Autodesk Fusion 360 part; units mm, degrees
note: some values were not read from the file. Set by a fixed rule: which sketch regions a step uses.
(part 2 of 2)
sketch "Sketch19" plane through (0, 0, 50.8) normal (0, 0, 1) x (-1, 0, 0)
  line L0 (-511.175, 2670.175) -> (-609.6, 2670.175)
  arc A0 (-609.6, 2670.175) -> (-1344.8064, 2362.3425) centre (-609.6, 1638.3) ccw
  arc A1 (-2923.5196, 2352.9776) -> (-1344.8064, 2362.3425) centre (-2138.8294, 3144.3083) ccw
  arc A2 (-2923.5196, 2352.9776) -> (-2963.6689, 2390.6683) centre (-3632.2, 1638.3) ccw
  arc A3 (-2963.6689, 2390.6683) -> (-3715.5992, 2670.175) centre (-3671.2525, 1638.3) ccw
  line L1 (-3715.5992, 2670.175) -> (-3730.6249, 2670.175)
  line L2 (-3730.6249, 2670.175) -> (-3730.6249, 2438.5075)
  line L3 (-3730.6249, 2438.5075) -> (-3759.1999, 2438.5075)
  line L4 (-3759.1999, 2438.5075) -> (-3759.1999, 3251.2)
  line L5 (-3759.1999, 3251.2) -> (-3730.6249, 3251.2)
  line L6 (-3730.6249, 3251.2) -> (-3730.6249, 3019.425)
  line L7 (-3730.6249, 3019.425) -> (-3632.2, 3019.425)
  arc A4 (-2659.7206, 2619.009) -> (-3632.2, 3019.425) centre (-3632.2, 1638.3) ccw
  arc A5 (-2659.7206, 2619.009) -> (-1611.7429, 2625.2256) centre (-2138.8294, 3144.3083) ccw
  arc A6 (-609.6, 3044.825) -> (-1611.7429, 2625.2256) centre (-609.6, 1638.3) ccw
  line L8 (-609.6, 3044.825) -> (-511.175, 3044.825)
  line L9 (-511.175, 3044.825) -> (-511.175, 3276.173)
  line L10 (-511.175, 3276.173) -> (-482.6, 3276.173)
  line L11 (-482.6, 3276.173) -> (-482.6, 3044.825)
  line L12 (-482.6, 3044.825) -> (0, 3044.825)
  line L13 (0, 3044.825) -> (0, 3276.6)
  line L14 (0, 3276.6) -> (-609.6, 3276.6)
  arc A7 (-609.6, 3276.6) -> (-1776.8816, 2787.8567) centre (-609.6, 1638.3) ccw
  arc A8 (-2496.523, 2783.5878) -> (-1776.8816, 2787.8567) centre (-2138.8294, 3144.3083) ccw
  arc A9 (-2496.523, 2783.5878) -> (-3632.2, 3251.2) centre (-3632.2, 1638.3) ccw
  line L15 (-3632.2, 3251.2) -> (-4241.8, 3251.2)
  line L16 (-4241.8, 3251.2) -> (-4241.8, 2438.4)
  line L17 (-4241.8, 2438.4) -> (-3710.305, 2438.4)
  arc A10 (-3710.305, 838.2) -> (-3710.305, 2438.4) centre (-3671.2525, 1638.3) ccw
  line L18 (-3710.305, 838.2) -> (-3730.625, 838.2)
  line L19 (-3730.625, 838.2) -> (-3730.625, 276.225)
  line L20 (-511.175, 250.825) -> (-511.175, 838.2)
  line L21 (-511.175, 838.2) -> (-482.6, 838.2)
  line L22 (-482.6, 838.2) -> (-482.6, 606.425)
  line L23 (-482.6, 606.425) -> (0, 606.425)
  line L24 (0, 606.425) -> (0, 838.2)
  line L25 (0, 838.2) -> (-531.495, 838.2)
  arc A11 (-531.495, 2438.4) -> (-531.495, 838.2) centre (-570.5475, 1638.3) ccw
  line L26 (-531.495, 2438.4) -> (0, 2438.4)
  line L27 (0, 2438.4) -> (0, 2670.175)
  line L28 (0, 2670.175) -> (-482.6, 2670.175)
  line L29 (-482.6, 2670.175) -> (-482.6, 2438.6051)
  line L30 (-482.6, 2438.6051) -> (-511.175, 2438.6051)
  line L31 (-511.175, 2438.6051) -> (-511.175, 2670.175)
  circle A12 centre (-3302, 2420.0312) radius 16
  circle A13 centre (-914.4, 845.0683) radius 16
  circle A14 centre (-863.6, 3192.4811) radius 16
  line L32 (-4241.8, 2689.225) -> (-3710.305, 2689.225)
  line L33 (-4241.8, 2670.175) -> (-3710.305, 2670.175)
  line L34 (-3730.625, 276.225) -> (-3632.2, 276.225)
  arc A15 (-3632.2, 276.225) -> (-2673.1342, 671.118) centre (-3632.2, 1638.3) ccw
  arc A16 (-1598.1699, 664.7414) -> (-2673.1342, 671.118) centre (-2138.8294, 132.2917) ccw
  arc A17 (-1598.1699, 664.7414) -> (-609.6, 250.825) centre (-609.6, 1638.3) ccw
  line L35 (-609.6, 250.825) -> (-511.175, 250.825)
  dimension "d130" = -250.825
  dimension "d131" = -231.775
extrude "Extrude20" add sketch "Sketch19" along normal blind 0.0279 contours L4 L16 L32 L33
sketch "Sketch20" plane through (0, 0, 50.8) normal (0, 0, 1) x (-1, 0, 0)
  line L0 (-4241.8, 2689.225) -> (-3759.1999, 2689.225)
  line L1 (-3759.1999, 2689.225) -> (-3759.1999, 3251.2)
  line L2 (-3759.1999, 3251.2) -> (-3730.6249, 3251.2)
  line L3 (-3730.6249, 3251.2) -> (-3730.6249, 3019.425)
  line L4 (-3730.6249, 3019.425) -> (-3632.2, 3019.425)
  arc A0 (-2659.7206, 2619.009) -> (-3632.2, 3019.425) centre (-3632.2, 1638.3) ccw
  arc A1 (-2659.7206, 2619.009) -> (-1611.7429, 2625.2256) centre (-2138.8294, 3144.3083) ccw
  arc A2 (-609.6, 3044.825) -> (-1611.7429, 2625.2256) centre (-609.6, 1638.3) ccw
  line L5 (-609.6, 3044.825) -> (-511.175, 3044.825)
  line L6 (-511.175, 3044.825) -> (-511.175, 3276.173)
  line L7 (-511.175, 3276.173) -> (-482.6, 3276.173)
  line L8 (-482.6, 3276.173) -> (-482.6, 3044.825)
  line L9 (-482.6, 3044.825) -> (0, 3044.825)
  line L10 (0, 3044.825) -> (0, 3276.6)
  line L11 (0, 3276.6) -> (-609.6, 3276.6)
  arc A3 (-609.6, 3276.6) -> (-1776.8816, 2787.8567) centre (-609.6, 1638.3) ccw
  arc A4 (-2496.523, 2783.5878) -> (-1776.8816, 2787.8567) centre (-2138.8294, 3144.3083) ccw
  arc A5 (-2496.523, 2783.5878) -> (-3632.2, 3251.2) centre (-3632.2, 1638.3) ccw
  line L12 (-3632.2, 3251.2) -> (-4241.8, 3251.2)
  line L13 (-4241.8, 3251.2) -> (-4241.8, 2689.225)
  circle A6 centre (-863.6, 3192.4811) radius 16
  line L14 (-3632.2, 3000.375) -> (-4241.8, 3000.375)
  line L15 (-3632.2, 3019.425) -> (-4241.8, 3019.425)
  dimension "d134" = -250.825
  dimension "d135" = -231.775
extrude "Extrude21" add sketch "Sketch20" along normal blind 0.0279 contours L1 L13 L14 L15
sketch "Sketch21" plane through (0, 0, 50.8) normal (0, 0, 1) x (-1, 0, 0)
  line L0 (-3759.2, 25.4) -> (-3759.2, 838.2)
  line L1 (-3759.2, 838.2) -> (-4241.8, 838.2)
  line L2 (-4241.8, 838.2) -> (-4241.8, 25.4)
  line L3 (-4241.8, 25.4) -> (-3759.2, 25.4)
sketch "Sketch22" plane through (0, 0, 50.8) normal (0, 0, 1) x (-1, 0, 0)
sketch "Sketch23" plane through (0, 0, 50.8) normal (0, 0, 1) x (-1, 0, 0)
extrude "Extrude22" add sketch "Sketch14" along normal blind 0.2794 contours L13 A11 L24 A12 A13 A14 L26 A15 A17 | A13 A15 A16 A17 A18 | L10 A13 A17 L28 A18 L29
sketch "Sketch24" plane through (0, 0, 50.8) normal (0, 0, 1) x (-1, 0, 0)
  line L0 (-3759.2, 25.4) -> (-3759.2, 838.2)
  line L1 (-3759.2, 838.2) -> (-4241.8, 838.2)
  line L2 (-4241.8, 838.2) -> (-4241.8, 25.4)
  line L3 (-4241.8, 25.4) -> (-3759.2, 25.4)
  line L4 (-3759.2, 587.375) -> (-4241.8, 587.375)
  line L5 (-3759.2, 606.425) -> (-4241.8, 606.425)
  dimension "d142" = -250.825
  dimension "d143" = -231.775
extrude "Extrude23" add sketch "Sketch24" along normal blind 0.0279 contours L0 L2 L4 L5
sketch "Sketch25" plane through (0, 0, 50.8) normal (0, 0, 1) x (-1, 0, 0)
  line L0 (-3759.2, 587.375) -> (-4241.8, 587.375)
  line L1 (-4241.8, 587.375) -> (-4241.8, 25.4)
  line L2 (-4241.8, 25.4) -> (-3759.2, 25.4)
  line L3 (-3759.2, 25.4) -> (-3759.2, 587.375)
  line L4 (-4241.8, 276.225) -> (-3759.2, 276.225)
  line L5 (-4241.8, 257.175) -> (-3759.2, 257.175)
  dimension "d146" = -250.825
  dimension "d147" = -231.775
extrude "Extrude24" add sketch "Sketch25" along normal blind 0.0279 contours L1 L3 L4 L5
equation "d13 = ( 63 / 2 ) * 1 in"
equation "d23 = ( 78.5 / 2 ) * 1 in"
